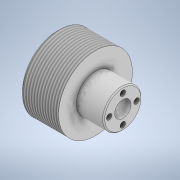
# Autodesk Inventor part: eixo parafuso
Saved by Autodesk Inventor 2022.1 (Build 261234020, 234B)
## iProperties
Created: 2023-08-25
Part Number: eixo parafuso
Material: Generic
Document SubType Name: Modeling
Designer: SENAI
Density: 1 g/cm^3
Appearance: Default
Author: SENAI
Autodesk Inventor part; units mm, degrees
ref_plane "YZ Plane" through (0, 0, 0) normal (1, 0, 0) x (0, 1, 0)
ref_plane "XZ Plane" through (0, 0, 0) normal (0, 1, 0) x (-1, 0, 0)
ref_plane "XY Plane" through (0, 0, 0) normal (0, 0, 1) x (1, 0, 0)
sketch "Sketch1" plane through (0, 0, 0) normal (0, 0, 1) x (1, 0, 0)
  line L0 (0, 0) -> (0, 33.75)
  line L1 (0, 33.75) -> (35, 33.75)
  line L2 (35, 17.5) -> (60, 17.5)
  line L3 (35, 33.75) -> (35, 17.5)
  line L4 (60, 17.5) -> (60, 0)
  line L5 (0, 0) -> (60, 0)
  dimension "d0" = 33.75
  dimension "d1" = 35
  dimension "d3" = 25
  constraints: 12 end point, 3 horizontal, 3 vertical
  measures "d0" distance of L0.start L0.end
  measures "d1" distance of L0.end L1.end
  measures "d3" distance of L2.start L2.end
revolve "Revolution1" add sketch "Sketch1" angle 360 about axis through (0, 0, 0) along (1, 0, 0)
thread "Thread1" size "M20x2.5" class "6g" standard "ISO Metric profile" full length
sketch "Sketch2" plane through (60, 0, 0) normal (1, 0, 0) x (0, 0, -1)
  circle A0 centre (0, 0) radius 7.5
  dimension "d7" = 15
  constraints: 1 centre point, 1 coincident
  measures "d7" diameter of A0
extrude "Extrusion1" cut sketch "Sketch2" against normal through all
chamfer "Chamfer1" distance 2 angle 45 1 edges at (0, -33.75, 0)
chamfer "Chamfer2" distance 1 angle 45 1 edges at (60, -17.5, 0)
sketch "Sketch3" plane through (0, 0, 0) normal (-1, 0, 0) x (0, 0, 1)
  circle A0 centre (0, 0) radius 26
  dimension "d16" = 52
  constraints: 1 centre point, 1 coincident
  measures "d16" diameter of A0
extrude "Extrusion2" cut sketch "Sketch3" against normal blind 18.5
sketch "Sketch4" plane through (18.5, 0, 0) normal (-1, 0, 0) x (0, 0, 1)
  circle A0 centre (0, 0) radius 10
  dimension "d19" = 20
  constraints: 1 centre point, 1 coincident
  measures "d19" diameter of A0
extrude "Extrusion3" cut sketch "Sketch4" against normal blind 3
sketch "Sketch5" plane through (60, 0, 0) normal (1, 0, 0) x (0, 0, -1)
  circle A0 centre (0, 0) radius 7.5 projected
  circle A1 centre (0, 12.5) radius 2.5
  circle A2 centre (12.5, 0) radius 2.5
  circle A3 centre (0, -12.5) radius 2.5
  circle A4 centre (-12.5, 0) radius 2.5
  dimension "d26" = 5
  dimension "d27" = 5
  dimension "d28" = 5
  dimension "d29" = 5
  constraints: 4 centre point
  measures "d26" diameter of A1
  measures "d27" diameter of A2
  measures "d28" diameter of A3
  measures "d29" diameter of A4
extrude "Extrusion4" cut sketch "Sketch5" against normal blind 27 contours A1 | A2 | A3 | A4
thread "Thread2" size "M5x0.8" class "6H" standard "ISO Metric profile" full length
thread "Thread3" size "M5x0.8" class "6H" standard "ISO Metric profile" full length
thread "Thread4" size "M5x0.8" class "6H" standard "ISO Metric profile" full length
thread "Thread5" size "M5x0.8" class "6H" standard "ISO Metric profile" full length
body "Solid1"
